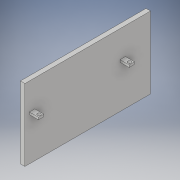
# Autodesk Inventor part: wire gaurd
Saved by Autodesk Inventor 2019 (Build 230136000, 136)
## iProperties
Created: 2020-02-06
Part Number: wire gaurd
Material: Generic
Document SubType Name: Modeling
Designer: User
Density: 1 g/cm^3
Appearance: Default
Author: User
Autodesk Inventor part; units mm, degrees
ref_plane "YZ Plane" through (0, 0, 0) normal (1, 0, 0) x (0, 1, 0)
ref_plane "XZ Plane" through (0, 0, 0) normal (0, 1, 0) x (-1, 0, 0)
ref_plane "XY Plane" through (0, 0, 0) normal (0, 0, 1) x (1, 0, 0)
sketch "Sketch1" plane through (0, 0, 0) normal (1, 0, 0) x (0, 1, 0)
  line L0 (0, 0) -> (101.6, 0)
  line L1 (101.6, 0) -> (101.6, 177.8)
  line L2 (101.6, 177.8) -> (0, 177.8)
  line L3 (0, 177.8) -> (0, 0)
  dimension "d0" = 101.6
  dimension "d1" = 177.8
  constraints: 8 end point, 2 parallel, 1 horizontal, 1 perpendicular
  measures "d0" distance between parallel lines of L3 L1
  measures "d1" distance between parallel lines of L2 L0
extrude "Extrusion1" add sketch "Sketch1" along normal blind 6.35
sketch "Sketch2" plane through (6.35, 0, 0) normal (1, 0, 0) x (0, 0, -1)
  line L0 (-35.56, 63.5) -> (-43.18, 63.5)
  line L1 (-43.18, 63.5) -> (-43.18, 60.325)
  line L2 (-43.18, 60.325) -> (-35.56, 60.325)
  line L3 (-35.56, 60.325) -> (-35.56, 63.5)
  line L4 (-163.83, 63.5) -> (-171.45, 63.5)
  line L5 (-171.45, 63.5) -> (-171.45, 60.325)
  line L6 (-171.45, 60.325) -> (-163.83, 60.325)
  line L7 (-163.83, 60.325) -> (-163.83, 63.5)
  line L8 (0, 101.6) -> (-177.8, 101.6) projected
  line L9 (0, 0) -> (0, 101.6) projected
  line L10 (-177.8, 101.6) -> (-177.8, 0) projected
  dimension "d4" = 38.1
  dimension "d5" = 38.1
  dimension "d6" = 3.175
  dimension "d7" = 3.175
  dimension "d11" = 128.27
  dimension "d12" = 7.62
  dimension "d13" = 7.62
  dimension "d30" = 6.35
  constraints: 16 end point, 4 parallel, 2 horizontal, 2 perpendicular
  measures "d4" distance between parallel lines of L8 L4
  measures "d5" distance between parallel lines of L8 L0
  measures "d6" distance between parallel lines of L0 L2
  measures "d7" distance between parallel lines of L4 L6
  measures "d11" distance between parallel lines of L5 L1
  measures "d12" distance between parallel lines of L7 L5
  measures "d13" distance between parallel lines of L1 L3
  measures "d30" distance between parallel lines of L10 L5
extrude "Extrusion2" add sketch "Sketch2" along normal blind 12.7
sketch "Sketch3" plane through (6.35, 63.5, 43.18) normal (0, 1, 0) x (1, 0, 0)
  line L0 (0, -128.27) -> (0, -120.65) projected
  line L1 (0, -128.27) -> (12.7, -128.27) projected
  line L2 (12.7, -120.65) -> (12.7, -128.27) projected
  line L3 (0, -120.65) -> (12.7, -120.65) projected
  line L4 (0, 0) -> (0, 7.62) projected
  line L5 (0, 0) -> (12.7, 0) projected
  line L6 (12.7, 7.62) -> (12.7, 0) projected
  line L7 (0, 7.62) -> (12.7, 7.62) projected
  point P0 (-6.35, 43.18)
  point P1 (9.525, 3.81)
  point P2 (9.525, -124.1806)
  dimension "d10" = 127.9906
  dimension "d15" = 3.81
  dimension "d16" = 12.7
  dimension "d17" = 7.62
  dimension "d28" = 3.175
  dimension "d29" = 3.175
  measures "d10" distance of point (9.525, -124.181) point (9.525, 3.81)
  measures "d15" distance from line of L7 point (9.525, 3.81)
  measures "d16" distance of L4.end L6.start
  measures "d17" distance of L6.start L5.end
  measures "d28" distance from line of L2 point (9.525, -124.181)
  measures "d29" distance from line of L6 point (9.525, 3.81)
hole "Hole1" at (15.875, 63.5, 167.3606) at (15.875, 63.5, 39.37) direction (0, -1, 0) diameter 4.7625 end through all
sketch "Sketch4" plane through (0, 0, 0) normal (-1, 0, 0) x (0, 0, 1)
  line L0 (4.3541, 3.3485) -> (4.3541, 0) construction
  line L1 (4.3541, 0) -> (0, 0) construction
  line L2 (0, 0) -> (0, 3.3485) construction
  line L3 (0, 3.3485) -> (4.3541, 3.3485) construction
  line L4 (1.7532, 2.2271) -> (0.412, 2.8001)
  line L5 (0.412, 2.8001) -> (0.412, 3.099)
  line L6 (0.412, 3.099) -> (1.7532, 2.7384)
  line L7 (1.7532, 2.7384) -> (1.7532, 2.2271)
  line L8 (2.8746, 2.363) -> (2.8746, 2.852)
  line L9 (2.8746, 2.852) -> (3.4575, 2.852)
  line L10 (3.4575, 2.852) -> (3.4575, 2.363)
  line L11 (3.4575, 2.363) -> (2.8746, 2.363)
  spline S0 degree 2 poles (2.341, 0.4808) (1.7087, 0.4808) (0.7504, 0.8859) (0.328, 1.244) knots 0 0 0 1 2 2 2
  line L12 (0.328, 1.244) -> (0.328, 1.7133)
  line L13 (0.328, 1.7133) -> (0.3477, 1.7133)
  spline S1 degree 2 poles (0.3477, 1.7133) (0.4885, 1.5553) (0.901, 1.2366) (1.148, 1.1181) knots 0 0 0 1 2 2 2
  spline S2 degree 2 poles (1.148, 1.1181) (1.4123, 0.9896) (2.0002, 0.8414) (2.341, 0.8414) knots 0 0 0 1 2 2 2
  spline S3 degree 2 poles (2.341, 0.8414) (2.6794, 0.8414) (3.2796, 0.9921) (3.5341, 1.1181) knots 0 0 0 1 2 2 2
  spline S4 degree 2 poles (3.5341, 1.1181) (3.7885, 1.2416) (4.1936, 1.5577) (4.3343, 1.7133) knots 0 0 0 1 2 2 2
  line L14 (4.3343, 1.7133) -> (4.3541, 1.7133)
  line L15 (4.3541, 1.7133) -> (4.3541, 1.244)
  spline S5 degree 2 poles (4.3541, 1.244) (3.9317, 0.8884) (2.9783, 0.4808) (2.341, 0.4808) knots 0 0 0 1 2 2 2
  constraints: 2 coincident, 2 other
extrude "Extrusion4" cut sketch "Sketch4" against normal blind 3.175
equation "\"d5\" = d4"
equation "\"d6\" = d7"
equation "\"d13\" = d12"
equation "\"d15\" = 0.5 * d17"
body "Solid1"
